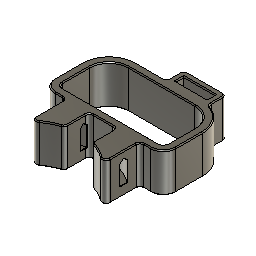
powerbox_mount_drillpress v1 (Autodesk Fusion 360 design; units mm, degrees)
Autodesk Fusion 360 part; units mm, degrees
sketch "Sketch1" plane through (0, 0, 0) normal (0, 0, 1) x (1, 0, 0)
  line L0 (-27.125, 20.875) -> (27.125, 20.875)
  line L1 (43.125, 4.875) -> (43.125, -16.875)
  line L2 (39.125, -20.875) -> (-39.125, -20.875)
  line L3 (-43.125, -16.875) -> (-43.125, 4.875)
  line L4 (-43.125, 20.875) -> (43.125, -20.875) construction
  line L5 (43.125, 20.875) -> (-43.125, -20.875) construction
  arc A0 (-27.125, 20.875) -> (-43.125, 4.875) centre (-27.125, 4.875) ccw
  arc A1 (43.125, 4.875) -> (27.125, 20.875) centre (27.125, 4.875) ccw
  arc A2 (-43.125, -16.875) -> (-39.125, -20.875) centre (-39.125, -16.875) ccw
  arc A3 (39.125, -20.875) -> (43.125, -16.875) centre (39.125, -16.875) ccw
  arc A4 (49.475, 4.875) -> (27.125, 27.225) centre (27.125, 4.875) ccw
  line L6 (-27.125, 27.225) -> (27.125, 27.225)
  arc A5 (-27.125, 27.225) -> (-49.475, 4.875) centre (-27.125, 4.875) ccw
  line L7 (-49.475, -16.875) -> (-49.475, 4.875)
  arc A6 (-49.475, -16.875) -> (-39.125, -27.225) centre (-39.125, -16.875) ccw
  line L8 (39.125, -27.225) -> (-39.125, -27.225)
  arc A7 (39.125, -27.225) -> (49.475, -16.875) centre (39.125, -16.875) ccw
  line L9 (49.475, 4.875) -> (49.475, -16.875)
  dimension "d1" = 86.25
  dimension "d2" = 41.75
  dimension "d3" = 16
  dimension "d4" = 4
  dimension "d5" = -6.35
  constraint horizontal L0
  constraint perpendicular L0 L1
  constraint parallel L0 L2
  constraint parallel L1 L3
  constraint coincident L4 origin
  constraint coincident L5 origin
  constraint coincident L4.start L3
  constraint coincident L4.start L0
  constraint tangent L3 A0
  constraint tangent L0 A0
  constraint coincident L5.start L0
  constraint coincident L5.start L1
  constraint tangent L0 A1
  constraint tangent L1 A1
  constraint equal A0 A1
  constraint coincident L5.end L2
  constraint coincident L5.end L3
  constraint tangent L2 A2
  constraint tangent L3 A2
  constraint coincident L4.end L2
  constraint coincident L4.end L1
  constraint tangent L2 A3
  constraint tangent L1 A3
  constraint equal A2 A3
  measures "d1" distance of L1 L3
  measures "d2" distance of L5.start L4.end
  measures "d3" radius of A0
  measures "d4" radius of A2
extrude "Extrude1" add sketch "Sketch1" along normal blind 31.75
sketch "Sketch2" plane through (0, 0, 31.75) normal (0, 0, 1) x (-1, 0, 0)
  arc A0 (43.125, 16.875) -> (39.125, 20.875) centre (39.125, 16.875) ccw
  line L0 (43.125, 16.875) -> (43.125, -4.875)
  arc A1 (27.125, -20.875) -> (43.125, -4.875) centre (27.125, -4.875) ccw
  line L1 (27.125, -20.875) -> (-27.125, -20.875)
  arc A2 (-43.125, -4.875) -> (-27.125, -20.875) centre (-27.125, -4.875) ccw
  line L2 (-43.125, -4.875) -> (-43.125, 16.875)
  arc A3 (-39.125, 20.875) -> (-43.125, 16.875) centre (-39.125, 16.875) ccw
  line L3 (-39.125, 20.875) -> (39.125, 20.875)
  arc A4 (27.125, -27.225) -> (49.475, -4.875) centre (27.125, -4.875) ccw
  line L4 (49.475, -4.875) -> (49.475, 16.875)
  arc A5 (49.475, 16.875) -> (39.125, 27.225) centre (39.125, 16.875) ccw
  line L5 (39.125, 27.225) -> (-39.125, 27.225)
  arc A6 (-39.125, 27.225) -> (-49.475, 16.875) centre (-39.125, 16.875) ccw
  line L6 (-49.475, 16.875) -> (-49.475, -4.875)
  arc A7 (-49.475, -4.875) -> (-27.125, -27.225) centre (-27.125, -4.875) ccw
  line L7 (-27.125, -27.225) -> (27.125, -27.225)
  circle A8 centre (0, 88.9) radius 42.8625
  line L8 (0, 88.9) -> (11.0936, 47.498)
  line L9 (0, 88.9) -> (30.3084, 58.5916)
  line L10 (0, 88.9) -> (-11.0936, 47.498)
  line L11 (0, 88.9) -> (-30.3084, 58.5916)
  line L12 (30.3084, 58.5916) -> (30.3084, 27.225)
  line L13 (-30.3084, 58.5916) -> (-30.3084, 27.225)
  line L14 (11.0936, 47.498) -> (11.0936, 27.225)
  line L15 (-11.0936, 47.498) -> (-11.0936, 27.225)
  dimension "d8" = 85.725
  dimension "d9" = 105
  dimension "d10" = 30
  dimension "d11" = 30
  dimension "d12" = 88.9
  constraint vertical origin A8.centre
  constraint coincident A8.centre L8.start
  constraint coincident A8 L8.end
  constraint coincident A8 L9.end
  constraint coincident A8 L10.end
  constraint coincident A8 L11.end
  constraint perpendicular L9 L11
  constraint coincident L5 L12.end
  constraint perpendicular L5 L12
  constraint coincident L5 L13.end
  constraint perpendicular L5 L13
  constraint coincident L5 L14.end
  constraint perpendicular L5 L14
  constraint coincident L5 L15.end
  constraint perpendicular L5 L15
  measures "d8" diameter of A8
  measures "d9" angle of L5 L10
  measures "d10" angle of L8 L10
  measures "d11" angle of L10 L11
  measures "d12" distance of origin A8.centre
extrude "Extrude2" add sketch "Sketch2" against normal blind 31.75 contours L5 A8 L12 L14 | L5 A8 L13 L15
sketch "Sketch3" plane through (0, 0, 0) normal (1, 0, 0) x (0, 1, 0)
  line L0 (-81.28, 36.1936) -> (-81.28, -23.5155)
  line L1 (-28.0988, 23.8125) -> (-32.8612, 23.8125)
  line L2 (-32.8612, 23.8125) -> (-32.8612, 7.9375)
  line L3 (-32.8612, 7.9375) -> (-28.0987, 7.9375)
  line L4 (-28.0988, 7.9375) -> (-28.0988, 23.8125)
  line L5 (-30.48, 23.8125) -> (-30.48, 7.9375) construction
  line L6 (-32.8612, 23.8125) -> (-30.48, 26.1937)
  line L7 (-30.48, 26.1937) -> (-28.0988, 23.8125)
  dimension "d17" = 81.28
  dimension "d18" = 15.875
  dimension "d19" = 4.7625
  dimension "d20" = 7.9375
  dimension "d21" = 50.8
  dimension "d23" = 45
  constraint vertical L0
  constraint horizontal L1
  constraint vertical L2
  constraint horizontal L3
  constraint vertical L4
  constraint midpoint L1 L5.start
  constraint midpoint L3 L5.end
  constraint equal L6 L7
  measures "d17" distance of origin L0
  measures "d18" distance of L1.end L2.end
  measures "d19" distance of L2.end L4.start
  measures "d20" distance of origin L3
  measures "d21" distance of L0 L5
  measures "d23" angle of L1 L6
revolve "Revolve1" cut sketch "Sketch3" angle 360 about axis through (0, -81.28, 36.1936) along (0, 0, -1)
fillet "Fillet1" radius 3.175 8 edges at (11.0936, -47.498, 15.875) (11.0936, -27.225, 15.875) (30.3084, -58.5916, 15.875) (30.3084, -27.225, 15.875) (-11.0936, -47.498, 15.875) (-11.0936, -27.225, 15.875) (-30.3084, -58.5916, 15.875) (-30.3084, -27.225, 15.875)
chamfer "Chamfer1" distance 0.254 angle 45 24 edges at (-30.3084, -39.0629, 25.0238) (-30.3084, -42.0342, 24.9803) (-30.3084, -37.5805, 15.875) (-30.3084, -40.5505, 7.9375) (-30.3084, -43.5205, 15.875) (30.3084, -37.5805, 15.875) (30.3084, -39.0629, 25.0238) (30.3084, -42.0342, 24.9803) (30.3084, -43.5205, 15.875) (30.3084, -40.5505, 7.9375) (-11.038, -29.8085, 24.352) (-11.0936, -31.0571, 25.5602) (-11.0936, -32.9423, 24.9881) (-11.0936, -34.1493, 15.875) (-11.0936, -32.2746, 7.9375) (-11.0363, -29.7995, 7.9375) (-10.8665, -29.2208, 15.875) (11.038, -29.8085, 24.352) (11.0936, -31.0571, 25.5602) (11.0936, -32.9423, 24.9881) (11.0936, -34.1493, 15.875) (10.8665, -29.2208, 15.875) (11.0936, -32.2746, 7.9375) (11.0363, -29.7995, 7.9375)
sketch "Sketch4" plane through (0, 0, 31.75) normal (0, 0, 1) x (-1, 0, 0)
  arc A0 (43.125, 16.875) -> (39.125, 20.875) centre (39.125, 16.875) ccw
  line L0 (43.125, 16.875) -> (43.125, -4.875)
  arc A1 (27.125, -20.875) -> (43.125, -4.875) centre (27.125, -4.875) ccw
  line L1 (27.125, -20.875) -> (-27.125, -20.875)
  arc A2 (-43.125, -4.875) -> (-27.125, -20.875) centre (-27.125, -4.875) ccw
  line L2 (-43.125, -4.875) -> (-43.125, 16.875)
  arc A3 (-39.125, 20.875) -> (-43.125, 16.875) centre (-39.125, 16.875) ccw
  line L3 (-39.125, 20.875) -> (39.125, 20.875)
  arc A4 (30.3084, 51.7082) -> (25.2621, 54.2731) centre (27.1334, 51.7082) ccw
  arc A5 (13.2846, 48.1481) -> (25.2621, 54.2731) centre (0, 88.9) ccw
  arc A6 (13.2846, 48.1481) -> (11.0936, 45.1295) centre (14.2686, 45.1295) ccw
  line L4 (11.0936, 45.1295) -> (11.0936, 30.4)
  arc A7 (7.9186, 27.225) -> (11.0936, 30.4) centre (7.9186, 30.4) ccw
  line L5 (7.9186, 27.225) -> (-7.9186, 27.225)
  arc A8 (-11.0936, 30.4) -> (-7.9186, 27.225) centre (-7.9186, 30.4) ccw
  line L6 (-11.0936, 30.4) -> (-11.0936, 45.1295)
  arc A9 (-11.0936, 45.1295) -> (-13.2846, 48.1481) centre (-14.2686, 45.1295) ccw
  arc A10 (-25.2621, 54.2731) -> (-13.2846, 48.1481) centre (0, 88.9) ccw
  arc A11 (-25.2621, 54.2731) -> (-30.3084, 51.7082) centre (-27.1334, 51.7082) ccw
  line L7 (-30.3084, 51.7082) -> (-30.3084, 30.4)
  arc A12 (-33.4834, 27.225) -> (-30.3084, 30.4) centre (-33.4834, 30.4) ccw
  line L8 (-33.4834, 27.225) -> (-39.125, 27.225)
  arc A13 (-39.125, 27.225) -> (-49.475, 16.875) centre (-39.125, 16.875) ccw
  line L9 (-49.475, 16.875) -> (-49.475, -4.875)
  arc A14 (-49.475, -4.875) -> (-27.125, -27.225) centre (-27.125, -4.875) ccw
  line L10 (-27.125, -27.225) -> (27.125, -27.225)
  arc A15 (27.125, -27.225) -> (49.475, -4.875) centre (27.125, -4.875) ccw
  line L11 (49.475, -4.875) -> (49.475, 16.875)
  arc A16 (49.475, 16.875) -> (39.125, 27.225) centre (39.125, 16.875) ccw
  line L12 (39.125, 27.225) -> (33.4834, 27.225)
  arc A17 (30.3084, 30.4) -> (33.4834, 27.225) centre (33.4834, 30.4) ccw
  line L13 (30.3084, 30.4) -> (30.3084, 51.7082)
  line L14 (-27.7, -30.4) -> (-2.3, -30.4)
  line L15 (-2.3, -30.4) -> (-2.3, -36.75)
  line L16 (-2.3, -36.75) -> (-27.7, -36.75)
  line L17 (-27.7, -36.75) -> (-27.7, -30.4)
  line L18 (-15, -30.4) -> (-15, -36.75) construction
  line L19 (2.4625, -41.5125) -> (-32.4625, -41.5125)
  line L20 (-32.4625, -41.5125) -> (-32.4625, -25.6375)
  line L21 (-32.4625, -25.6375) -> (2.4625, -25.6375)
  line L22 (2.4625, -25.6375) -> (2.4625, -41.5125)
  dimension "d26" = 15
  dimension "d27" = 6.35
  dimension "d28" = 3.175
  dimension "d29" = 25.4
  dimension "d30" = -4.7625
  constraint horizontal L14
  constraint vertical L15
  constraint horizontal L16
  constraint vertical L17
  constraint midpoint L14 L18.start
  constraint midpoint L16 L18.end
  measures "d26" distance of origin L18
  measures "d27" distance of L14.end L15.end
  measures "d28" distance of L10 L14
  measures "d29" distance of L15.end L16.end
extrude "Extrude3" add sketch "Sketch4" against normal blind 31.75 contours A14 L10 L19 L20 L22
fillet "Fillet2" radius 3.175 4 edges at (-2.4625, 27.225, 15.875) (-2.4625, 41.5125, 15.875) (32.4625, 41.5125, 15.875) (32.4625, 26.5783, 15.875)
chamfer "Chamfer3" distance 0.7937 angle 45 2 faces at (-17.4985, -35.3098, 31.75) (-17.4985, -35.3098, 0)
